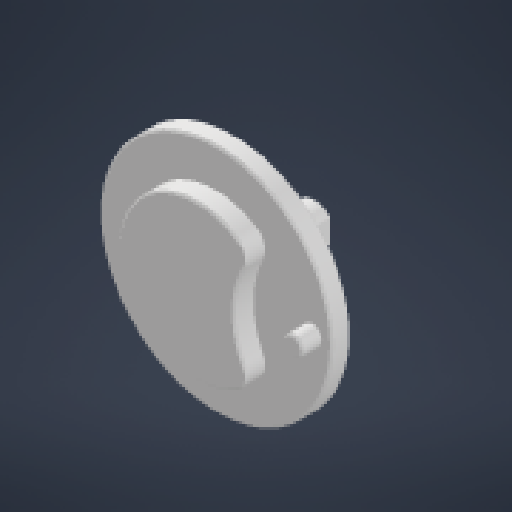
# Autodesk Inventor part: geniva1
Saved by Autodesk Inventor 2026.3 (Build 303398000, 398)
## iProperties
Created: 2026-04-30
Part Number: geniva1
Material: Generic
Document SubType Name: Modeling
Designer: frede
Density: 1 g/cm^3
Appearance: Default
Author: frede
Autodesk Inventor part; units mm, degrees
ref_plane "YZ Plane" through (0, 0, 0) normal (1, 0, 0) x (0, 1, 0)
ref_plane "XZ Plane" through (0, 0, 0) normal (0, 1, 0) x (-1, 0, 0)
ref_plane "XY Plane" through (0, 0, 0) normal (0, 0, 1) x (1, 0, 0)
sketch "Sketch2" plane through (0, 0, 0) normal (0, 0, 1) x (1, 0, 0)
  circle A0 centre (0, 0) radius 30
  dimension "d21" = 60
  constraints: 1 centre point, 1 coincident
  measures "d21" diameter of A0
extrude "Extrusion1" add sketch "Sketch2" along normal blind 5
sketch "Sketch4" plane through (0, 0, 5) normal (0, 0, 1) x (1, 0, 0)
  circle A0 centre (0, 0) radius 20
  circle A1 centre (25, 0) radius 2.5
  circle A2 centre (35.36, 0) radius 25.5
  point P0 (14.1414, -14.1429)
  point P1 (14.1414, 14.1429)
  dimension "d36" = 40
  dimension "d37" = 5
  dimension "d39" = 51
  dimension "d42" = 35.36
  constraints: 3 centre point, 1 coincident
  measures "d36" diameter of A0
  measures "d37" diameter of A1
  measures "d39" diameter of A2
  measures "d42" distance of point (0, 0) A2.centre
extrude "Extrusion3" add sketch "Sketch4" along normal blind 5.1 contours A2 A0 | A1 picked at (0.0752, -0.8246)
chamfer "Chamfer1" distance 0.5 angle 45 5 edges at (-20, 0, 10.1) (9.86, 0, 10.1) (22.5, 0, 10.1) (-30, 0, 5) (-30, 0, 0)
sketch "Sketch7" plane through (0, 0, 0) normal (0, 0, -1) x (-1, 0, 0)
  circle A0 centre (0, 0) radius 7
  dimension "d52" = 14
  constraints: 1 centre point, 1 coincident
  measures "d52" diameter of A0
extrude "Extrusion6" add sketch "Sketch7" along normal blind 1
sketch "Sketch8" plane through (0, 0, -1) normal (0, 0, -1) x (-1, 0, 0)
  circle A0 centre (0, 0) radius 5
  dimension "d55" = 10
  constraints: 1 centre point, 1 coincident
  measures "d55" diameter of A0
extrude "Extrusion7" add sketch "Sketch8" along normal blind 20
fillet "Fillet3" radius 0.8 2 edges at (7, 0, 0) (5, 0, -1)
chamfer "Chamfer2" distance 0.2 angle 45 1 edges at (7, 0, -1)
sketch "Sketch9" plane through (0, 0, -21) normal (0, 0, -1) x (-1, 0, 0)
  arc A0 (-4, 3) -> (-4, -3) centre (0, 0) ccw
  line L0 (-4, -3) -> (-4, 3)
  circle A1 centre (0, 0) radius 6.8 projected
  constraints: 2 end point, 2 point on circle, 1 centre point, 1 coincident, 1 vertical
extrude "Extrusion8" cut sketch "Sketch9" against normal blind 10 contours L0 A0
chamfer "Chamfer3" distance 0.5 angle 45 3 edges at (4, 0, -21) (-1.5811, -4.7434, -21) (-1.5811, 4.7434, -21)
fillet "Fillet4" radius 5 2 edges at (14.1414, 14.1429, 7.3) (14.1414, -14.1429, 7.3)
body "Solid1"
